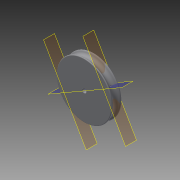
# Autodesk Inventor part: Big_Spool
Saved by Autodesk Inventor 2015 (Build 190159000, 159)
## iProperties
Created: 2014-11-21
Part Number: Big_Spool
Material: Generic
Document SubType Name: Modeling
Designer: Ryan
Density: 1 g/cm^3
Appearance: Default
Author: Ryan
Autodesk Inventor part; units mm, degrees
ref_plane "YZ Plane" through (0, 0, 0) normal (1, 0, 0) x (0, 1, 0)
ref_plane "XZ Plane" through (0, 0, 0) normal (0, 1, 0) x (-1, 0, 0)
ref_plane "XY Plane" through (0, 0, 0) normal (0, 0, 1) x (1, 0, 0)
sketch "Sketch1" plane through (0, 0, 0) normal (0, 0, 1) x (1, 0, 0)
  circle A0 centre (0, 0) radius 20
  dimension "d0" = 40
  constraints: 1 centre point, 1 coincident
  measures "d0" diameter of A0
extrude "Extrusion1" add sketch "Sketch1" along normal blind 1
sketch "Sketch2" plane through (0, 0, 1) normal (0, 0, 1) x (1, 0, 0)
  circle A0 centre (0, 0) radius 17.5
  dimension "d3" = 35
  constraints: 1 centre point, 1 coincident
  measures "d3" diameter of A0
extrude "Extrusion2" add sketch "Sketch2" along normal blind 5
sketch "Sketch3" plane through (0, 0, 6) normal (0, 0, 1) x (1, 0, 0)
  circle A0 centre (0, 0) radius 20
  dimension "d6" = 40
  constraints: 1 centre point, 1 coincident
  measures "d6" diameter of A0
extrude "Extrusion3" add sketch "Sketch3" along normal blind 1
fillet "Fillet1" radius 2.5 1 edges at (-17.5, 0, 6)
fillet "Fillet2" radius 2.5 1 edges at (-17.5, 0, 1)
fillet "Fillet3" radius 2.5 2 edges at (-19.9999, 0, 6) (-20, 0, 6)
fillet "Fillet4" radius 2.5 2 edges at (-19.9999, 0, 1) (-20, 0, 1)
sketch "Sketch4" plane through (0, 0, 0) normal (0, 0, -1) x (-1, 0, 0)
  line L0 (14.65, 0) -> (-14.65, 0) construction
  line L1 (-7.325, -12.6873) -> (7.325, 12.6873) construction
  line L2 (7.325, -12.6873) -> (-7.325, 12.6873) construction
  circle A0 centre (14.65, 0) radius 2.4
  circle A1 centre (7.325, -12.6873) radius 2.4
  circle A2 centre (-7.325, -12.6873) radius 2.4
  circle A3 centre (-14.65, 0) radius 2.4
  circle A4 centre (-7.325, 12.6873) radius 2.4
  circle A5 centre (7.325, 12.6873) radius 2.4
  line L3 (15.2712, -2.3182) -> (7.5833, -4.3782)
  line L4 (7.5833, -4.3782) -> (9.6432, -12.0661)
  line L5 (5.6279, -14.3843) -> (0, -8.7564)
  line L6 (0, -8.7564) -> (-5.6279, -14.3843)
  line L7 (-9.6432, -12.0661) -> (-7.5833, -4.3782)
  line L8 (-7.5833, -4.3782) -> (-15.2712, -2.3182)
  line L9 (-15.2712, 2.3182) -> (-7.5833, 4.3782)
  line L10 (-7.5833, 4.3782) -> (-9.6432, 12.0661)
  line L11 (-5.6279, 14.3843) -> (0, 8.7564)
  line L12 (0, 0) -> (0, -1.6279) construction
  line L13 (0, 0) -> (7.5833, 4.3782) construction
  line L14 (0, 0) -> (7.5833, -4.3782) construction
  line L15 (0, 0) -> (0, -8.7564) construction
  line L16 (0, 0) -> (0, 8.7564) construction
  line L17 (0, 0) -> (-7.5833, 4.3782) construction
  line L18 (0, 0) -> (-7.5833, -4.3782) construction
  line L19 (0, 8.7564) -> (5.6279, 14.3843)
  line L20 (9.6432, 12.0661) -> (7.5833, 4.3782)
  line L21 (7.5833, 4.3782) -> (15.2712, 2.3182)
  dimension "d13" = 4.8
  dimension "d14" = 4.8
  dimension "d15" = 4.8
  dimension "d16" = 4.8
  dimension "d17" = 4.8
  dimension "d18" = 4.8
  dimension "d22" = 34.1
  dimension "d23" = 34.1
  dimension "d24" = 60
  constraints: 44 end point, 12 point on circle, 12 tangent, 6 centre point, 6 symmetric about line, 5 coincident, 5 midpoint, 3 collinear, 2 perpendicular, 2 vertical, 1 horizontal, 1 point on line, 6 other
  measures "d13" diameter of A0
  measures "d14" diameter of A1
  measures "d15" diameter of A2
  measures "d16" diameter of A3
  measures "d17" diameter of A4
  measures "d18" diameter of A5
  measures "d24" angle of L1 L0
extrude "Extrusion4" cut sketch "Sketch4" against normal blind 5.5
sketch "Sketch5" plane through (0, 0, 0) normal (0, 0, -1) x (-1, 0, 0)
  line L0 (9.7266, 5.6156) -> (16.2733, 3.8614)
  line L1 (16.2733, 3.8614) -> (11.4808, 12.1624)
  line L2 (11.4808, 12.1624) -> (9.7266, 5.6156)
  line L3 (0, 11.2313) -> (4.7926, 16.0238)
  line L4 (4.7926, 16.0238) -> (-4.7926, 16.0238)
  line L5 (-4.7926, 16.0238) -> (0, 11.2313)
  line L6 (-9.7266, 5.6156) -> (-16.2733, 3.8614)
  line L7 (-16.2733, 3.8614) -> (-11.4808, 12.1624)
  line L8 (-11.4808, 12.1624) -> (-9.7266, 5.6156)
  line L9 (-9.7266, -5.6156) -> (-16.2733, -3.8614)
  line L10 (-16.2733, -3.8614) -> (-11.4808, -12.1624)
  line L11 (-11.4808, -12.1624) -> (-9.7266, -5.6156)
  line L12 (0, -11.2313) -> (4.7926, -16.0238)
  line L13 (4.7926, -16.0238) -> (-4.7926, -16.0238)
  line L14 (-4.7926, -16.0238) -> (0, -11.2313)
  line L15 (9.7266, -5.6156) -> (11.4808, -12.1624)
  line L16 (11.4808, -12.1624) -> (16.2733, -3.8614)
  line L17 (16.2733, -3.8614) -> (9.7266, -5.6156)
  line L18 (0, 8.7564) -> (5.6279, 14.3843) projected
  line L19 (-5.6279, 14.3843) -> (0, 8.7564) projected
  line L20 (-7.5833, 4.3782) -> (-9.6432, 12.0661) projected
  line L21 (-15.2712, 2.3182) -> (-7.5833, 4.3782) projected
  line L22 (-7.5833, -4.3782) -> (-15.2712, -2.3182) projected
  line L23 (-9.6432, -12.0661) -> (-7.5833, -4.3782) projected
  line L24 (0, -8.7564) -> (-5.6279, -14.3843) projected
  line L25 (5.6279, -14.3843) -> (0, -8.7564) projected
  line L26 (7.5833, -4.3782) -> (9.6432, -12.0661) projected
  line L27 (15.2712, -2.3182) -> (7.5833, -4.3782) projected
  line L28 (7.5833, 4.3782) -> (15.2712, 2.3182) projected
  line L29 (9.6432, 12.0661) -> (7.5833, 4.3782) projected
  line L30 (0, 0) -> (9.7266, 5.6156) construction
  line L31 (0, 0) -> (9.7266, -5.6156) construction
  line L32 (0, 0) -> (0, -11.2313) construction
  line L33 (9.7266, 5.6156) -> (13.877, 8.0119) construction
  line L34 (9.7266, -5.6156) -> (13.877, -8.0119) construction
  line L35 (0, -11.2313) -> (0, -16.0238) construction
  line L36 (-9.7266, -5.6156) -> (-13.877, -8.0119) construction
  line L37 (-9.7266, 5.6156) -> (-13.877, 8.0119) construction
  line L38 (0, 11.2313) -> (0, 16.0238) construction
  line L39 (0, 11.2313) -> (0, 0) construction
  line L40 (-9.7266, 5.6156) -> (0, 0) construction
  line L41 (-9.7266, -5.6156) -> (0, 0) construction
  arc A0 (4.7926, 16.0238) -> (-4.7926, 16.0238) centre (0, 0) ccw
  arc A1 (-11.4808, 12.1624) -> (-16.2733, 3.8614) centre (0, 0) ccw
  arc A2 (-16.2733, -3.8614) -> (-11.4808, -12.1624) centre (0, 0) ccw
  arc A3 (-4.7926, -16.0238) -> (4.7926, -16.0238) centre (0, 0) ccw
  arc A4 (11.4808, -12.1624) -> (16.2733, -3.8614) centre (0, 0) ccw
  arc A5 (16.2733, 3.8614) -> (11.4808, 12.1624) centre (0, 0) ccw
  dimension "d50" = 1.75
  constraints: 60 end point, 15 parallel, 12 point on circle, 10 equal length, 6 centre point, 6 midpoint, 3 perpendicular, 3 point on line, 2 vertical, 1 coincident, 10 other
  measures "d50" distance between parallel lines of L25 L12
extrude "Extrusion5" cut sketch "Sketch5" against normal blind 5.5
ref_plane "Work Plane1" through (9.7266, 5.6156, 0) normal (0.5, -0.8660254, 0) x (0, 0, 1)
ref_plane "Work Plane2" through (11.4808, 12.1624, 0) normal (0.8660254, 0.5, 0) x (0, 0, 1)
ref_plane "Work Plane3" through (-16.2733, -3.8614, 0) normal (0.8660254, 0.5, 0) x (0, 0, 1)
sketch "Sketch6" plane through (11.4808, 12.1624, 0) normal (0.8660254, 0.5, 0) x (0, 0, 1)
  line L0 (0, 4.7926) -> (5.5, 4.7926) projected
  circle A0 centre (3.5, 4.7926) radius 0.5
  line L1 (0, 4.7926) -> (3.5, 4.7926)
  line L2 (7, 4.7926) -> (3.5, 4.7926)
  dimension "d33" = 1
  constraints: 4 end point, 3 collinear, 1 centre point, 1 point on line
  measures "d33" diameter of A0
extrude "Extrusion6" cut sketch "Sketch6" along normal blind 5.5
sketch "Sketch7" plane through (-16.2733, -3.8614, 0) normal (0.8660254, 0.5, 0) x (0, 0, 1)
  circle A0 centre (3.5, 4.7926) radius 0.5
  line L0 (0, 4.7926) -> (3.5, 4.7926)
  line L1 (3.5, 4.7926) -> (7, 4.7926)
  line L2 (7, 9.5851) -> (7, 0)
  line L3 (0, 9.5851) -> (0, 0)
  point P0 (0, 4.7926)
  dimension "d36" = 1
  constraints: 8 end point, 2 midpoint, 2 vertical, 1 centre point, 1 collinear, 1 horizontal, 1 point on line
  measures "d36" diameter of A0
extrude "Extrusion7" cut sketch "Sketch7" against normal blind 5.5
fillet "Fillet5" radius 0.5 18 edges at (16.2733, -3.8614, 2.75) (9.7266, -5.6156, 2.75) (11.4808, -12.1624, 2.75) (16.2733, 3.8614, 2.75) (11.4808, 12.1624, 2.75) (9.7266, 5.6156, 2.75) (4.7926, 16.0238, 2.75) (-4.7926, 16.0238, 2.75) (0, 11.2313, 2.75) (-9.7266, 5.6156, 2.75) (-11.4808, 12.1624, 2.75) (-16.2733, 3.8614, 2.75) (-16.2733, -3.8614, 2.75) (-9.7266, -5.6156, 2.75) (-11.4808, -12.1624, 2.75) (0, -11.2313, 2.75) (4.7926, -16.0238, 2.75) (-4.7926, -16.0238, 2.75)
fillet "Fillet7" radius 1 6 edges at (7.5833, 4.3782, 2.75) (0, 8.7564, 2.75) (-7.5833, 4.3782, 2.75) (-7.5833, -4.3782, 2.75) (7.5833, -4.3782, 2.75) (0, -8.7564, 2.75)
fillet "Fillet6" [suppressed]
sketch "Sketch8" plane through (0, 0, 7) normal (0, 0, 1) x (1, 0, 0)
  circle A0 centre (0, 0) radius 1.55
  dimension "d41" = 3.1
  constraints: 1 centre point, 1 coincident
  measures "d41" diameter of A0
extrude "Extrusion8" cut sketch "Sketch8" against normal blind 5.5
sketch "Sketch9" plane through (0, 0, 5.5) normal (0, 0, -1) x (-1, 0, 0)
  circle A0 centre (0, 0) radius 4
  dimension "d44" = 8
  constraints: 1 centre point, 1 coincident
  measures "d44" diameter of A0
extrude "Extrusion9" cut sketch "Sketch9" against normal blind 0.5
fillet "Fillet8" radius 0.5 2 edges at (-20, 0, 7) (-20, 0, 0)
sketch "Sketch10" plane through (0, 0, 6) normal (0, 0, -1) x (-1, 0, 0)
  circle A0 centre (0, 0) radius 2.45
  circle A1 centre (0, 0) radius 1.55 projected
  dimension "d53" = 4.9
  constraints: 1 centre point, 1 coincident
  measures "d53" diameter of A0
extrude "Extrusion10" add sketch "Sketch10" along normal blind 1.5
chamfer "Chamfer2" distance 0.25 angle 45 1 edges at (2.45, 0, 4.5)
body "Solid1"
